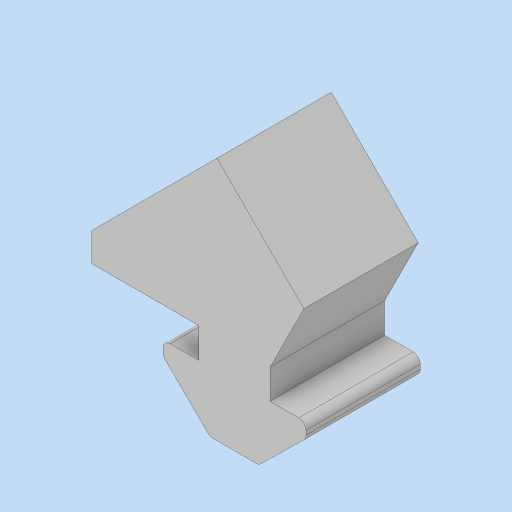
# Autodesk Inventor part: Profil-ElBoardHold
Saved by Autodesk Inventor 2024 (Build 280153000, 153)
## iProperties
Created: 2023-05-09
Part Number: Profil-ElBoardHold
Material: Generic
Document SubType Name: Modeling
Designer: Karbosch
Mass: 1.05374 g
Surface Area: 8.18959 cm^2
Volume: 1.05374 cm^3
Density: 1 g/cm^3
Appearance: Default
Author: Karbosch
Autodesk Inventor part; units mm, degrees
ref_plane "YZ Plane" through (0, 0, 0) normal (1, 0, 0) x (0, 1, 0)
ref_plane "XZ Plane" through (0, 0, 0) normal (0, 1, 0) x (-1, 0, 0)
ref_plane "XY Plane" through (0, 0, 0) normal (0, 0, 1) x (1, 0, 0)
sketch "Sketch1" plane through (0, 0, 0) normal (0, 0, 1) x (1, 0, 0)
  arc A0 (-5, -2.9) -> (-4.8506, -3.2565) centre (-4.5, -2.9) ccw
  line L0 (-5, -2.6) -> (-5, -2.9)
  arc A1 (-4.5, -2.1) -> (-5, -2.6) centre (-4.5, -2.6) ccw
  line L1 (-4.8506, -3.2565) -> (-1.8506, -6.2065)
  arc A2 (-1.8506, -6.2065) -> (-1.5, -6.35) centre (-1.5, -5.85) ccw
  line L2 (-1.5, -6.35) -> (1.5, -6.35)
  line L3 (4.5, -2.1) -> (-4.5, -2.1)
  arc A3 (1.5, -6.35) -> (1.8506, -6.2065) centre (1.5, -5.85) ccw
  line L4 (4.8506, -3.2565) -> (1.8506, -6.2065)
  arc A4 (5, -2.6) -> (4.5, -2.1) centre (4.5, -2.6) ccw
  arc A5 (4.8506, -3.2565) -> (5, -2.9) centre (4.5, -2.9) ccw
  line L5 (5, -2.6) -> (5, -2.9)
  line L6 (-2.5, 0) -> (2.5, 0)
  line L7 (-2.5, 0) -> (-2.5, -2.1)
  line L8 (2.5, 0) -> (2.5, -2.1)
  point P0 (0, -6.35)
  point P1 (0, 0)
  point P2 (0, -2.1)
  point P3 (0, 0)
  dimension "d9" = 4.25
  dimension "d10" = 10
  dimension "d12" = 0.3
  dimension "d13" = 9
  dimension "d14" = 3
  dimension "d17" = 2.1
  dimension "d18" = 5
  constraints: 18 end point, 12 point on circle, 12 tangent, 6 centre point, 5 equal radius, 5 vertical alignment, 3 horizontal, 3 midpoint, 2 perpendicular, 2 point on line, 2 vertical, 1 coincident, 1 equal length, 1 horizontal alignment
  measures "d9" distance between parallel lines of L2 L3
  measures "d10" distance between parallel lines of L5 L0
  measures "d12" distance of A4.centre A5.centre
  measures "d13" distance of A4.centre A1.centre
  measures "d14" distance of A3.centre A2.centre
  measures "d17" distance of point (0, -2.1) point (0, 0)
  measures "d18" distance of L6.start L6.end
extrude "Extrusion1" add sketch "Sketch1" along normal blind 8
sketch "Sketch2" plane through (0, 0, 0) normal (0, 0, -1) x (-1, 0, 0)
  line L0 (-2.5, 0) -> (2.5, 0) projected
  line L1 (2.5, 0) -> (12, 0)
  line L2 (-2.5, -2.1) -> (-2.5, 0) projected
  line L3 (12, 0) -> (3.3532, 8.6468)
  line L4 (-0.6066, 4.687) -> (2.0804, 2)
  line L5 (3.3532, 8.6468) -> (-0.6066, 4.687)
  line L6 (2.0804, 2) -> (6.0402, 5.9598)
  line L7 (10, 0) -> (10, 2)
  line L8 (3.3532, 8.6468) -> (1.2319, 10.7681)
  line L9 (1.2319, 10.7681) -> (-4.8492, 4.687)
  line L10 (-4.8492, 4.687) -> (-2.5, 0)
  point P0 (0, 0)
  dimension "d21" = 12
  dimension "d23" = 45
  dimension "d24" = 3.8
  dimension "d25" = 5.6
  dimension "d26" = 2
  dimension "d28" = 3
  dimension "d34" = 10
  constraints: 18 end point, 4 perpendicular, 3 point on line, 1 collinear, 1 horizontal, 1 horizontal alignment, 1 parallel
  measures "d21" distance of point (0, 0) L1.end
  measures "d23" angle of L1 L3
  measures "d24" distance of L4.start L4.end
  measures "d25" distance of L3.end L4.start
  measures "d26" distance from line of L0 L4.end
  measures "d28" distance of L3.end L8.end
  measures "d34" distance of point (0, 0) L7.start
extrude "Extrusion2" add sketch "Sketch2" against normal up to surface (8 mm away) contours L10 L9 L8 L5 L4 L6 L3 L7 L1 L0 | L3 L6 L4 L5
sketch "Sketch3" plane through (-1.2319, 10.7681, 0) normal (-0.7071, 0.7071, 0) x (-0.7071, -0.7071, 0)
  line L0 (12.4, 0) -> (12.4, 8) projected
  line L1 (6.8, 0) -> (3, 0)
  line L2 (12.4, 0) -> (0, 0) projected
  circle A0 centre (4.9, 4) radius 1.9
  point P0 (6.7431, 0)
  point P1 (12.4, 4)
  point P2 (4.9, 0)
  dimension "d31" = 3.8
  constraints: 2 end point, 2 midpoint, 1 centre point, 1 collinear, 1 horizontal alignment, 1 vertical alignment
  measures "d31" diameter of A0
extrude "Extrusion3" cut sketch "Sketch3" against normal blind 5.6
body "Solid1"
